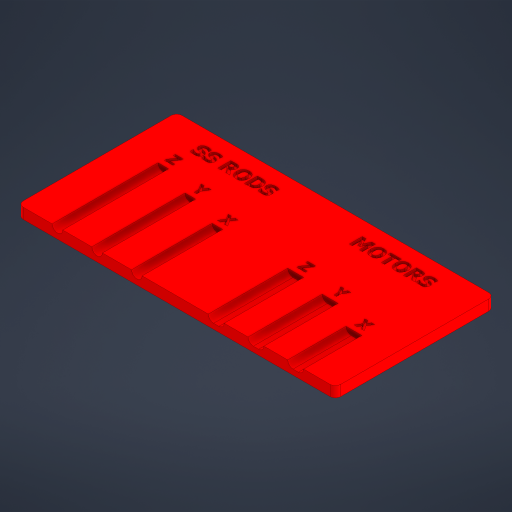
# Autodesk Inventor part: Rod_Motor_Lengths
Saved by Autodesk Inventor 2023.4 (Build 274418000, 418)
## iProperties
Created: 2024-09-24
Part Number: Rod_Motor_Lengths
Material: Generic
Document SubType Name: Modeling
Designer: xSibe
Density: 1 g/cm^3
Appearance: Plastic Red
Author: xSibe
Autodesk Inventor part; units mm, degrees
ref_plane "YZ Plane" through (0, 0, 0) normal (1, 0, 0) x (0, 1, 0)
ref_plane "XZ Plane" through (0, 0, 0) normal (0, 1, 0) x (-1, 0, 0)
ref_plane "XY Plane" through (0, 0, 0) normal (0, 0, 1) x (1, 0, 0)
sketch "Sketch1" plane through (0, 0, 0) normal (0, 1, 0) x (-1, 0, 0)
  line L0 (75, 37.5) -> (-75, 37.5)
  line L1 (-75, 37.5) -> (-75, -37.5)
  line L2 (-75, -37.5) -> (75, -37.5)
  line L3 (75, -37.5) -> (75, 37.5)
  line L4 (75, 37.5) -> (-75, -37.5) construction
  line L5 (-75, 37.5) -> (75, -37.5) construction
  line L6 (0, 37.5) -> (0, -37.5)
  line L7 (0, 37.5) -> (75, 37.5)
  line L8 (0, 37.5) -> (37.5, 37.5)
  line L9 (37.5, 37.5) -> (75, 37.5)
  line L10 (56.25, 37.5) -> (56.25, -12.5)
  line L11 (37.5, 37.5) -> (37.5, -6.5)
  line L12 (18.75, 37.5) -> (18.75, -0.5)
  line L13 (-18.75, 37.5) -> (-18.75, 0)
  line L14 (-37.5, 37.5) -> (-37.5, 2.5)
  line L15 (-56.25, 37.5) -> (-56.25, 10)
  line L16 (58.75, -12.5) -> (53.75, -12.5)
  line L17 (53.75, -12.5) -> (53.75, 37.5)
  line L18 (53.75, 37.5) -> (58.75, 37.5)
  line L19 (58.75, 37.5) -> (58.75, -12.5)
  line L20 (58.75, -12.5) -> (53.75, 37.5) construction
  line L21 (53.75, -12.5) -> (58.75, 37.5) construction
  line L22 (40, -6.5) -> (35, -6.5)
  line L23 (35, -6.5) -> (35, 37.5)
  line L24 (35, 37.5) -> (40, 37.5)
  line L25 (40, 37.5) -> (40, -6.5)
  line L26 (40, -6.5) -> (35, 37.5) construction
  line L27 (35, -6.5) -> (40, 37.5) construction
  line L28 (21.25, -0.5) -> (16.25, -0.5)
  line L29 (16.25, -0.5) -> (16.25, 37.5)
  line L30 (16.25, 37.5) -> (21.25, 37.5)
  line L31 (21.25, 37.5) -> (21.25, -0.5)
  line L32 (21.25, -0.5) -> (16.25, 37.5) construction
  line L33 (16.25, -0.5) -> (21.25, 37.5) construction
  line L34 (0, 37.5) -> (-75, 37.5)
  line L35 (-37.5, 37.5) -> (-75, 37.5)
  line L36 (-37.5, 37.5) -> (0, 37.5)
  line L37 (-15, 0) -> (-22.5, 0)
  line L38 (-22.5, 0) -> (-22.5, 37.5)
  line L39 (-22.5, 37.5) -> (-15, 37.5)
  line L40 (-15, 37.5) -> (-15, 0)
  line L41 (-15, 0) -> (-22.5, 37.5) construction
  line L42 (-22.5, 0) -> (-15, 37.5) construction
  line L43 (-33.75, 2.5) -> (-41.25, 2.5)
  line L44 (-41.25, 2.5) -> (-41.25, 37.5)
  line L45 (-41.25, 37.5) -> (-33.75, 37.5)
  line L46 (-33.75, 37.5) -> (-33.75, 2.5)
  line L47 (-33.75, 2.5) -> (-41.25, 37.5) construction
  line L48 (-41.25, 2.5) -> (-33.75, 37.5) construction
  line L49 (-52.5, 10) -> (-60, 10)
  line L50 (-60, 10) -> (-60, 37.5)
  line L51 (-60, 37.5) -> (-52.5, 37.5)
  line L52 (-52.5, 37.5) -> (-52.5, 10)
  line L53 (-52.5, 10) -> (-60, 37.5) construction
  line L54 (-60, 10) -> (-52.5, 37.5) construction
  point P0 (0, 0)
  point P1 (56.25, 12.5)
  point P2 (37.5, 15.5)
  point P3 (18.75, 18.5)
  point P4 (-18.75, 18.75)
  point P5 (-37.5, 20)
  point P6 (-56.25, 23.75)
  dimension "d0" = 150
  dimension "d1" = 75
  dimension "d2" = 50
  dimension "d3" = 44
  dimension "d4" = 38
  dimension "d5" = 37.5
  dimension "d6" = 35
  dimension "d7" = 27.5
  dimension "d8" = 5
  dimension "d9" = 5
  dimension "d10" = 5
  dimension "d11" = 7.5
  dimension "d12" = 7.5
  dimension "d13" = 7.5
  constraints: 110 end point, 28 midpoint, 14 parallel, 12 perpendicular, 7 horizontal, 6 point on line, 4 vertical, 3 collinear
  measures "d0" distance of L2.end L1.end
  measures "d1" distance of L1.end L0.end
  measures "d2" distance of L10.start L10.end
  measures "d3" distance of L8.end L11.end
  measures "d4" distance of L12.start L12.end
  measures "d5" distance of L13.start L13.end
  measures "d6" distance of L14.start L14.end
  measures "d7" distance of L15.start L15.end
  measures "d8" distance of L17.end L18.end
  measures "d9" distance of L23.end L24.end
  measures "d10" distance of L29.end L30.end
  measures "d11" distance of L38.end L39.end
  measures "d12" distance of L44.end L45.end
  measures "d13" distance of L50.end L51.end
extrude "Extrusion1" add sketch "Sketch1" along normal blind 5 contours L3 L2 L6 L0 L29 L28 L31 L23 L22 L25 L17 L16 L19 | L2 L1 L0 L50 L49 L52 L44 L43 L46 L38 L37 L40 L6
extrude "Extrusion2" add sketch "Sketch1" along normal blind 2.5
sketch "Sketch2" plane through (0, 5, 0) normal (0, 1, 0) x (1, 0, 0)
  line L0 (-75, -37.5) -> (-58.75, -37.5) projected
  line L1 (-58.75, -37.5) -> (-58.75, 12.5) projected
  line L2 (-58.75, 12.5) -> (-53.75, 12.5) projected
  line L3 (-53.75, 12.5) -> (-53.75, -37.5) projected
  line L4 (-53.75, -37.5) -> (-40, -37.5) projected
  line L5 (-40, -37.5) -> (-40, 6.5) projected
  line L6 (-40, 6.5) -> (-35, 6.5) projected
  line L7 (-35, 6.5) -> (-35, -37.5) projected
  line L8 (-35, -37.5) -> (-21.25, -37.5) projected
  line L9 (-21.25, -37.5) -> (-21.25, 0.5) projected
  line L10 (-21.25, 0.5) -> (-16.25, 0.5) projected
  line L11 (-16.25, 0.5) -> (-16.25, -37.5) projected
  line L12 (-16.25, -37.5) -> (15, -37.5) projected
  line L13 (15, -37.5) -> (15, 0) projected
  line L14 (15, 0) -> (22.5, 0) projected
  line L15 (22.5, 0) -> (22.5, -37.5) projected
  line L16 (22.5, -37.5) -> (33.75, -37.5) projected
  line L17 (33.75, -37.5) -> (33.75, -2.5) projected
  line L18 (33.75, -2.5) -> (41.25, -2.5) projected
  line L19 (41.25, -2.5) -> (41.25, -37.5) projected
  line L20 (41.25, -37.5) -> (52.5, -37.5) projected
  line L21 (52.5, -37.5) -> (52.5, -10) projected
  line L22 (52.5, -10) -> (60, -10) projected
  line L23 (60, -10) -> (60, -37.5) projected
  line L24 (60, -37.5) -> (75, -37.5) projected
  line L25 (75, -37.5) -> (75, 37.5) projected
  line L26 (75, 37.5) -> (-75, 37.5) projected
  line L27 (-75, 37.5) -> (-75, -37.5) projected
  line L28 (-75, 37.5) -> (0, 37.5)
  line L29 (0, 37.5) -> (0, 0)
  line L30 (0, 0) -> (-75, 0)
  line L31 (-75, 0) -> (-75, 37.5)
  line L32 (0, 37.5) -> (75, 37.5)
  line L33 (75, 37.5) -> (75, 0)
  line L34 (75, 0) -> (0, 0)
  line L35 (0, 0) -> (0, 37.5)
  line L36 (-37.5, 37.5) -> (-37.5, 27.5)
  line L37 (-62.5, 22.5) -> (-12.5, 22.5)
  line L38 (-12.5, 22.5) -> (-12.5, 32.5)
  line L39 (-12.5, 32.5) -> (-62.5, 32.5)
  line L40 (-62.5, 32.5) -> (-62.5, 22.5)
  line L41 (-62.5, 22.5) -> (-12.5, 32.5) construction
  line L42 (-12.5, 22.5) -> (-62.5, 32.5) construction
  line L43 (37.5, 37.5) -> (37.5, 27.5)
  line L44 (12.5, 22.5) -> (62.5, 22.5)
  line L45 (62.5, 22.5) -> (62.5, 32.5)
  line L46 (62.5, 32.5) -> (12.5, 32.5)
  line L47 (12.5, 32.5) -> (12.5, 22.5)
  line L48 (12.5, 22.5) -> (62.5, 32.5) construction
  line L49 (62.5, 22.5) -> (12.5, 32.5) construction
  line L50 (-62.5, 32.5) -> (-12.5, 32.5) construction
  line L51 (-12.5, 32.5) -> (-12.5, 22.5) construction
  line L52 (-12.5, 22.5) -> (-62.5, 22.5) construction
  line L53 (-62.5, 22.5) -> (-62.5, 32.5) construction
  line L54 (12.5, 32.5) -> (62.5, 32.5) construction
  line L55 (62.5, 32.5) -> (62.5, 22.5) construction
  line L56 (62.5, 22.5) -> (12.5, 22.5) construction
  line L57 (12.5, 22.5) -> (12.5, 32.5) construction
  line L58 (-58.75, 20) -> (-53.75, 20) construction
  line L59 (-53.75, 20) -> (-53.75, 12.5) construction
  line L60 (-53.75, 12.5) -> (-58.75, 12.5) construction
  line L61 (-58.75, 12.5) -> (-58.75, 20) construction
  line L62 (-40, 14) -> (-35, 14) construction
  line L63 (-35, 14) -> (-35, 6.5) construction
  line L64 (-35, 6.5) -> (-40, 6.5) construction
  line L65 (-40, 6.5) -> (-40, 14) construction
  line L66 (-21.25, 8) -> (-16.25, 8) construction
  line L67 (-16.25, 8) -> (-16.25, 0.5) construction
  line L68 (-16.25, 0.5) -> (-21.25, 0.5) construction
  line L69 (-21.25, 0.5) -> (-21.25, 8) construction
  line L70 (15, 7.5) -> (22.5, 7.5) construction
  line L71 (22.5, 7.5) -> (22.5, 0) construction
  line L72 (22.5, 0) -> (15, 0) construction
  line L73 (15, 0) -> (15, 7.5) construction
  line L74 (33.75, 5) -> (41.25, 5) construction
  line L75 (41.25, 5) -> (41.25, -2.5) construction
  line L76 (41.25, -2.5) -> (33.75, -2.5) construction
  line L77 (33.75, -2.5) -> (33.75, 5) construction
  line L78 (52.5, -2.5) -> (60, -2.5) construction
  line L79 (60, -2.5) -> (60, -10) construction
  line L80 (60, -10) -> (52.5, -10) construction
  line L81 (52.5, -10) -> (52.5, -2.5) construction
  spline S0 degree 2 poles (-53.6348, 24.3412) (-54.3368, 24.3412) (-55.3947, 24.6131) (-55.8494, 24.8109) knots 0 0 0 1 2 2 2
  line L82 (-55.8494, 24.8109) -> (-55.8494, 26.2642)
  line L83 (-55.8494, 26.2642) -> (-55.711, 26.2642)
  spline S1 degree 2 poles (-55.711, 26.2642) (-55.2513, 25.8737) (-54.1489, 25.4535) (-53.6299, 25.4535) knots 0 0 0 1 2 2 2
  spline S2 degree 2 poles (-53.6299, 25.4535) (-53.4964, 25.4535) (-53.0664, 25.5128) (-52.9378, 25.5721) knots 0 0 0 1 2 2 2
  spline S3 degree 2 poles (-52.9378, 25.5721) (-52.7797, 25.6413) (-52.5572, 25.8934) (-52.5572, 26.0961) knots 0 0 0 1 2 2 2
  spline S4 degree 2 poles (-52.5572, 26.0961) (-52.5572, 26.3284) (-52.9181, 26.6152) (-53.1652, 26.6794) knots 0 0 0 1 2 2 2
  spline S5 degree 2 poles (-53.1652, 26.6794) (-53.4767, 26.7635) (-54.1835, 26.9068) (-54.495, 27.0156) knots 0 0 0 1 2 2 2
  spline S6 degree 2 poles (-54.495, 27.0156) (-55.2019, 27.2627) (-55.8148, 28.108) (-55.8148, 28.7408) knots 0 0 0 1 2 2 2
  spline S7 degree 2 poles (-55.8148, 28.7408) (-55.8148, 29.5959) (-54.3665, 30.6588) (-53.2789, 30.6588) knots 0 0 0 1 2 2 2
  spline S8 degree 2 poles (-53.2789, 30.6588) (-52.7352, 30.6588) (-51.6575, 30.4363) (-51.2324, 30.2485) knots 0 0 0 1 2 2 2
  line L84 (-51.2324, 30.2485) -> (-51.2324, 28.8545)
  line L85 (-51.2324, 28.8545) -> (-51.3659, 28.8545)
  spline S9 degree 2 poles (-51.3659, 28.8545) (-51.707, 29.1461) (-52.6857, 29.5465) (-53.1998, 29.5465) knots 0 0 0 1 2 2 2
  spline S10 degree 2 poles (-53.1998, 29.5465) (-53.4025, 29.5465) (-53.7189, 29.4872) (-53.8968, 29.4081) knots 0 0 0 1 2 2 2
  spline S11 degree 2 poles (-53.8968, 29.4081) (-54.0402, 29.3438) (-54.2478, 29.0868) (-54.2478, 28.9286) knots 0 0 0 1 2 2 2
  spline S12 degree 2 poles (-54.2478, 28.9286) (-54.2478, 28.6913) (-53.9166, 28.4194) (-53.4421, 28.3107) knots 0 0 0 1 2 2 2
  spline S13 degree 2 poles (-53.4421, 28.3107) (-53.1356, 28.2415) (-52.5671, 28.108) (-52.2408, 27.9943) knots 0 0 0 1 2 2 2
  spline S14 degree 2 poles (-52.2408, 27.9943) (-51.6081, 27.762) (-50.9902, 26.9908) (-50.9902, 26.3581) knots 0 0 0 1 2 2 2
  spline S15 degree 2 poles (-50.9902, 26.3581) (-50.9902, 25.4485) (-52.4188, 24.3412) (-53.6348, 24.3412) knots 0 0 0 1 2 2 2
  spline S16 degree 2 poles (-48.3208, 24.3412) (-49.0228, 24.3412) (-50.0806, 24.6131) (-50.5354, 24.8109) knots 0 0 0 1 2 2 2
  line L86 (-50.5354, 24.8109) -> (-50.5354, 26.2642)
  line L87 (-50.5354, 26.2642) -> (-50.397, 26.2642)
  spline S17 degree 2 poles (-50.397, 26.2642) (-49.9373, 25.8737) (-48.8349, 25.4535) (-48.3159, 25.4535) knots 0 0 0 1 2 2 2
  spline S18 degree 2 poles (-48.3159, 25.4535) (-48.1824, 25.4535) (-47.7524, 25.5128) (-47.6238, 25.5721) knots 0 0 0 1 2 2 2
  spline S19 degree 2 poles (-47.6238, 25.5721) (-47.4656, 25.6413) (-47.2432, 25.8934) (-47.2432, 26.0961) knots 0 0 0 1 2 2 2
  spline S20 degree 2 poles (-47.2432, 26.0961) (-47.2432, 26.3284) (-47.6041, 26.6152) (-47.8512, 26.6794) knots 0 0 0 1 2 2 2
  spline S21 degree 2 poles (-47.8512, 26.6794) (-48.1626, 26.7635) (-48.8695, 26.9068) (-49.181, 27.0156) knots 0 0 0 1 2 2 2
  spline S22 degree 2 poles (-49.181, 27.0156) (-49.8878, 27.2627) (-50.5008, 28.108) (-50.5008, 28.7408) knots 0 0 0 1 2 2 2
  spline S23 degree 2 poles (-50.5008, 28.7408) (-50.5008, 29.5959) (-49.0524, 30.6588) (-47.9649, 30.6588) knots 0 0 0 1 2 2 2
  spline S24 degree 2 poles (-47.9649, 30.6588) (-47.4212, 30.6588) (-46.3435, 30.4363) (-45.9184, 30.2485) knots 0 0 0 1 2 2 2
  line L88 (-45.9184, 30.2485) -> (-45.9184, 28.8545)
  line L89 (-45.9184, 28.8545) -> (-46.0519, 28.8545)
  spline S25 degree 2 poles (-46.0519, 28.8545) (-46.3929, 29.1461) (-47.3717, 29.5465) (-47.8858, 29.5465) knots 0 0 0 1 2 2 2
  spline S26 degree 2 poles (-47.8858, 29.5465) (-48.0885, 29.5465) (-48.4049, 29.4872) (-48.5828, 29.4081) knots 0 0 0 1 2 2 2
  spline S27 degree 2 poles (-48.5828, 29.4081) (-48.7262, 29.3438) (-48.9338, 29.0868) (-48.9338, 28.9286) knots 0 0 0 1 2 2 2
  spline S28 degree 2 poles (-48.9338, 28.9286) (-48.9338, 28.6913) (-48.6026, 28.4194) (-48.128, 28.3107) knots 0 0 0 1 2 2 2
  spline S29 degree 2 poles (-48.128, 28.3107) (-47.8216, 28.2415) (-47.2531, 28.108) (-46.9268, 27.9943) knots 0 0 0 1 2 2 2
  spline S30 degree 2 poles (-46.9268, 27.9943) (-46.2941, 27.762) (-45.6762, 26.9908) (-45.6762, 26.3581) knots 0 0 0 1 2 2 2
  spline S31 degree 2 poles (-45.6762, 26.3581) (-45.6762, 25.4485) (-47.1048, 24.3412) (-48.3208, 24.3412) knots 0 0 0 1 2 2 2
  line L90 (-36.7981, 24.45) -> (-38.6617, 24.45)
  line L91 (-38.6617, 24.45) -> (-40.3572, 26.6893)
  line L92 (-40.3572, 26.6893) -> (-40.9109, 26.6893)
  line L93 (-40.9109, 26.6893) -> (-40.9109, 24.45)
  line L94 (-40.9109, 24.45) -> (-42.4334, 24.45)
  line L95 (-42.4334, 24.45) -> (-42.4334, 30.55)
  line L96 (-42.4334, 30.55) -> (-39.9815, 30.55)
  spline S32 degree 2 poles (-39.9815, 30.55) (-39.4724, 30.55) (-38.721, 30.4215) (-38.3997, 30.2237) knots 0 0 0 1 2 2 2
  spline S33 degree 2 poles (-38.3997, 30.2237) (-38.0734, 30.0161) (-37.6878, 29.3686) (-37.6878, 28.8742) knots 0 0 0 1 2 2 2
  spline S34 degree 2 poles (-37.6878, 28.8742) (-37.6878, 28.1772) (-38.3206, 27.3023) (-38.8495, 27.0452) knots 0 0 0 1 2 2 2
  line L97 (-38.8495, 27.0452) -> (-36.7981, 24.45)
  spline S35 degree 2 poles (-39.2598, 28.6814) (-39.2598, 28.9138) (-39.4378, 29.245) (-39.6404, 29.334) knots 0 0 0 1 2 2 2
  spline S36 degree 2 poles (-39.6404, 29.334) (-39.7838, 29.3933) (-40.1348, 29.4279) (-40.3968, 29.4279) knots 0 0 0 1 2 2 2
  line L98 (-40.3968, 29.4279) -> (-40.9109, 29.4279)
  line L99 (-40.9109, 29.4279) -> (-40.9109, 27.7867)
  line L100 (-40.9109, 27.7867) -> (-40.4709, 27.7867)
  spline S37 degree 2 poles (-40.4709, 27.7867) (-40.1545, 27.7867) (-39.7047, 27.8658) (-39.5515, 27.9894) knots 0 0 0 1 2 2 2
  spline S38 degree 2 poles (-39.5515, 27.9894) (-39.4032, 28.108) (-39.2598, 28.4244) (-39.2598, 28.6814) knots 0 0 0 1 2 2 2
  spline S39 degree 2 poles (-30.792, 27.5) (-30.792, 26.017) (-32.3738, 24.3215) (-33.7481, 24.3215) knots 0 0 0 1 2 2 2
  spline S40 degree 2 poles (-33.7481, 24.3215) (-35.1272, 24.3215) (-36.6992, 26.0368) (-36.6992, 27.5) knots 0 0 0 1 2 2 2
  spline S41 degree 2 poles (-36.6992, 27.5) (-36.6992, 28.9682) (-35.1272, 30.6785) (-33.7481, 30.6785) knots 0 0 0 1 2 2 2
  spline S42 degree 2 poles (-33.7481, 30.6785) (-32.3738, 30.6785) (-30.792, 28.978) (-30.792, 27.5) knots 0 0 0 1 2 2 2
  spline S43 degree 2 poles (-32.3738, 27.5) (-32.3738, 28.0487) (-32.5963, 28.8149) (-32.7891, 29.0571) knots 0 0 0 1 2 2 2
  spline S44 degree 2 poles (-32.7891, 29.0571) (-32.9818, 29.3092) (-33.4762, 29.5267) (-33.7431, 29.5267) knots 0 0 0 1 2 2 2
  spline S45 degree 2 poles (-33.7431, 29.5267) (-34.0249, 29.5267) (-34.4846, 29.3241) (-34.6972, 29.067) knots 0 0 0 1 2 2 2
  spline S46 degree 2 poles (-34.6972, 29.067) (-34.885, 28.8297) (-35.1173, 28.0438) (-35.1173, 27.5) knots 0 0 0 1 2 2 2
  spline S47 degree 2 poles (-35.1173, 27.5) (-35.1173, 26.9365) (-34.8949, 26.195) (-34.7021, 25.9429) knots 0 0 0 1 2 2 2
  spline S48 degree 2 poles (-34.7021, 25.9429) (-34.5093, 25.6908) (-34.01, 25.4733) (-33.7431, 25.4733) knots 0 0 0 1 2 2 2
  spline S49 degree 2 poles (-33.7431, 25.4733) (-33.4712, 25.4733) (-32.967, 25.7056) (-32.7841, 25.9528) knots 0 0 0 1 2 2 2
  spline S50 degree 2 poles (-32.7841, 25.9528) (-32.5864, 26.2197) (-32.3738, 26.9266) (-32.3738, 27.5) knots 0 0 0 1 2 2 2
  spline S51 degree 2 poles (-24.4399, 27.4951) (-24.4399, 26.6399) (-25.1863, 25.2953) (-25.7548, 24.9344) knots 0 0 0 1 2 2 2
  spline S52 degree 2 poles (-25.7548, 24.9344) (-26.2293, 24.628) (-27.3465, 24.45) (-27.9743, 24.45) knots 0 0 0 1 2 2 2
  line L101 (-27.9743, 24.45) -> (-29.8824, 24.45)
  line L102 (-29.8824, 24.45) -> (-29.8824, 30.55)
  line L103 (-29.8824, 30.55) -> (-27.9941, 30.55)
  spline S53 degree 2 poles (-27.9941, 30.55) (-27.3515, 30.55) (-26.2293, 30.3869) (-25.735, 30.0705) knots 0 0 0 1 2 2 2
  spline S54 degree 2 poles (-25.735, 30.0705) (-25.1369, 29.6849) (-24.4399, 28.3799) (-24.4399, 27.4951) knots 0 0 0 1 2 2 2
  spline S55 degree 2 poles (-26.0118, 27.5049) (-26.0118, 28.108) (-26.4271, 28.9682) (-26.8522, 29.2104) knots 0 0 0 1 2 2 2
  spline S56 degree 2 poles (-26.8522, 29.2104) (-27.1636, 29.3784) (-27.8458, 29.413) (-28.3203, 29.413) knots 0 0 0 1 2 2 2
  line L104 (-28.3203, 29.413) -> (-28.35, 29.413)
  line L105 (-28.35, 29.413) -> (-28.35, 25.5919)
  line L106 (-28.35, 25.5919) -> (-28.3203, 25.5919)
  spline S57 degree 2 poles (-28.3203, 25.5919) (-27.8062, 25.5919) (-27.0994, 25.6265) (-26.778, 25.8292) knots 0 0 0 1 2 2 2
  spline S58 degree 2 poles (-26.778, 25.8292) (-26.4023, 26.0665) (-26.0118, 26.9019) (-26.0118, 27.5049) knots 0 0 0 1 2 2 2
  spline S59 degree 2 poles (-21.6469, 24.3412) (-22.3489, 24.3412) (-23.4067, 24.6131) (-23.8615, 24.8109) knots 0 0 0 1 2 2 2
  line L107 (-23.8615, 24.8109) -> (-23.8615, 26.2642)
  line L108 (-23.8615, 26.2642) -> (-23.7231, 26.2642)
  spline S60 degree 2 poles (-23.7231, 26.2642) (-23.2634, 25.8737) (-22.161, 25.4535) (-21.642, 25.4535) knots 0 0 0 1 2 2 2
  spline S61 degree 2 poles (-21.642, 25.4535) (-21.5085, 25.4535) (-21.0784, 25.5128) (-20.9499, 25.5721) knots 0 0 0 1 2 2 2
  spline S62 degree 2 poles (-20.9499, 25.5721) (-20.7917, 25.6413) (-20.5693, 25.8934) (-20.5693, 26.0961) knots 0 0 0 1 2 2 2
  spline S63 degree 2 poles (-20.5693, 26.0961) (-20.5693, 26.3284) (-20.9301, 26.6152) (-21.1773, 26.6794) knots 0 0 0 1 2 2 2
  spline S64 degree 2 poles (-21.1773, 26.6794) (-21.4887, 26.7635) (-22.1956, 26.9068) (-22.507, 27.0156) knots 0 0 0 1 2 2 2
  spline S65 degree 2 poles (-22.507, 27.0156) (-23.2139, 27.2627) (-23.8269, 28.108) (-23.8269, 28.7408) knots 0 0 0 1 2 2 2
  spline S66 degree 2 poles (-23.8269, 28.7408) (-23.8269, 29.5959) (-22.3785, 30.6588) (-21.291, 30.6588) knots 0 0 0 1 2 2 2
  spline S67 degree 2 poles (-21.291, 30.6588) (-20.7472, 30.6588) (-19.6696, 30.4363) (-19.2445, 30.2485) knots 0 0 0 1 2 2 2
  line L109 (-19.2445, 30.2485) -> (-19.2445, 28.8545)
  line L110 (-19.2445, 28.8545) -> (-19.378, 28.8545)
  spline S68 degree 2 poles (-19.378, 28.8545) (-19.719, 29.1461) (-20.6978, 29.5465) (-21.2119, 29.5465) knots 0 0 0 1 2 2 2
  spline S69 degree 2 poles (-21.2119, 29.5465) (-21.4146, 29.5465) (-21.731, 29.4872) (-21.9089, 29.4081) knots 0 0 0 1 2 2 2
  spline S70 degree 2 poles (-21.9089, 29.4081) (-22.0523, 29.3438) (-22.2599, 29.0868) (-22.2599, 28.9286) knots 0 0 0 1 2 2 2
  spline S71 degree 2 poles (-22.2599, 28.9286) (-22.2599, 28.6913) (-21.9287, 28.4194) (-21.4541, 28.3107) knots 0 0 0 1 2 2 2
  spline S72 degree 2 poles (-21.4541, 28.3107) (-21.1476, 28.2415) (-20.5792, 28.108) (-20.2529, 27.9943) knots 0 0 0 1 2 2 2
  spline S73 degree 2 poles (-20.2529, 27.9943) (-19.6202, 27.762) (-19.0023, 26.9908) (-19.0023, 26.3581) knots 0 0 0 1 2 2 2
  spline S74 degree 2 poles (-19.0023, 26.3581) (-19.0023, 25.4485) (-20.4309, 24.3412) (-21.6469, 24.3412) knots 0 0 0 1 2 2 2
  line L111 (-54.2443, 15) -> (-58.2071, 15)
  line L112 (-58.2071, 15) -> (-58.2071, 15.936)
  line L113 (-58.2071, 15.936) -> (-55.9015, 19.0478)
  line L114 (-55.9015, 19.0478) -> (-58.0855, 19.0478)
  line L115 (-58.0855, 19.0478) -> (-58.0855, 20)
  line L116 (-58.0855, 20) -> (-54.378, 20)
  line L117 (-54.378, 20) -> (-54.378, 19.0478)
  line L118 (-54.378, 19.0478) -> (-56.6754, 15.9522)
  line L119 (-56.6754, 15.9522) -> (-54.2443, 15.9522)
  line L120 (-54.2443, 15.9522) -> (-54.2443, 15)
  line L121 (-35.1925, 14) -> (-36.9186, 11.0867)
  line L122 (-36.9186, 11.0867) -> (-36.9186, 9)
  line L123 (-36.9186, 9) -> (-38.1746, 9)
  line L124 (-38.1746, 9) -> (-38.1746, 11.0259)
  line L125 (-38.1746, 11.0259) -> (-39.9291, 14)
  line L126 (-39.9291, 14) -> (-38.4988, 14)
  line L127 (-38.4988, 14) -> (-37.5223, 12.2172)
  line L128 (-37.5223, 12.2172) -> (-36.5782, 14)
  line L129 (-36.5782, 14) -> (-35.1925, 14)
  line L130 (-16.3959, 3) -> (-17.8464, 3)
  line L131 (-17.8464, 3) -> (-18.8108, 4.5924)
  line L132 (-18.8108, 4.5924) -> (-19.7954, 3)
  line L133 (-19.7954, 3) -> (-21.1852, 3)
  line L134 (-21.1852, 3) -> (-19.5604, 5.5162)
  line L135 (-19.5604, 5.5162) -> (-21.1203, 8)
  line L136 (-21.1203, 8) -> (-19.6698, 8)
  line L137 (-19.6698, 8) -> (-18.7662, 6.4887)
  line L138 (-18.7662, 6.4887) -> (-17.8383, 8)
  line L139 (-17.8383, 8) -> (-16.4485, 8)
  line L140 (-16.4485, 8) -> (-18.0166, 5.5689)
  line L141 (-18.0166, 5.5689) -> (-16.3959, 3)
  line L142 (20.7557, 2.5) -> (16.7929, 2.5)
  line L143 (16.7929, 2.5) -> (16.7929, 3.436)
  line L144 (16.7929, 3.436) -> (19.0985, 6.5478)
  line L145 (19.0985, 6.5478) -> (16.9145, 6.5478)
  line L146 (16.9145, 6.5478) -> (16.9145, 7.5)
  line L147 (16.9145, 7.5) -> (20.622, 7.5)
  line L148 (20.622, 7.5) -> (20.622, 6.5478)
  line L149 (20.622, 6.5478) -> (18.3246, 3.4522)
  line L150 (18.3246, 3.4522) -> (20.7557, 3.4522)
  line L151 (20.7557, 3.4522) -> (20.7557, 2.5)
  line L152 (25.8833, 24.45) -> (24.3608, 24.45)
  line L153 (24.3608, 24.45) -> (24.3608, 28.4936)
  line L154 (24.3608, 28.4936) -> (23.2535, 25.8835)
  line L155 (23.2535, 25.8835) -> (22.2055, 25.8835)
  line L156 (22.2055, 25.8835) -> (21.0982, 28.4936)
  line L157 (21.0982, 28.4936) -> (21.0982, 24.45)
  line L158 (21.0982, 24.45) -> (19.6548, 24.45)
  line L159 (19.6548, 24.45) -> (19.6548, 30.55)
  line L160 (19.6548, 30.55) -> (21.4195, 30.55)
  line L161 (21.4195, 30.55) -> (22.774, 27.5395)
  line L162 (22.774, 27.5395) -> (24.1186, 30.55)
  line L163 (24.1186, 30.55) -> (25.8833, 30.55)
  line L164 (25.8833, 30.55) -> (25.8833, 24.45)
  spline S75 degree 2 poles (32.7001, 27.5) (32.7001, 26.017) (31.1182, 24.3215) (29.744, 24.3215) knots 0 0 0 1 2 2 2
  spline S76 degree 2 poles (29.744, 24.3215) (28.3648, 24.3215) (26.7929, 26.0368) (26.7929, 27.5) knots 0 0 0 1 2 2 2
  spline S77 degree 2 poles (26.7929, 27.5) (26.7929, 28.9682) (28.3648, 30.6785) (29.744, 30.6785) knots 0 0 0 1 2 2 2
  spline S78 degree 2 poles (29.744, 30.6785) (31.1182, 30.6785) (32.7001, 28.978) (32.7001, 27.5) knots 0 0 0 1 2 2 2
  spline S79 degree 2 poles (31.1182, 27.5) (31.1182, 28.0487) (30.8958, 28.8149) (30.703, 29.0571) knots 0 0 0 1 2 2 2
  spline S80 degree 2 poles (30.703, 29.0571) (30.5102, 29.3092) (30.0159, 29.5267) (29.7489, 29.5267) knots 0 0 0 1 2 2 2
  spline S81 degree 2 poles (29.7489, 29.5267) (29.4672, 29.5267) (29.0075, 29.3241) (28.7949, 29.067) knots 0 0 0 1 2 2 2
  spline S82 degree 2 poles (28.7949, 29.067) (28.607, 28.8297) (28.3747, 28.0438) (28.3747, 27.5) knots 0 0 0 1 2 2 2
  spline S83 degree 2 poles (28.3747, 27.5) (28.3747, 26.9365) (28.5972, 26.195) (28.79, 25.9429) knots 0 0 0 1 2 2 2
  spline S84 degree 2 poles (28.79, 25.9429) (28.9827, 25.6908) (29.482, 25.4733) (29.7489, 25.4733) knots 0 0 0 1 2 2 2
  spline S85 degree 2 poles (29.7489, 25.4733) (30.0208, 25.4733) (30.525, 25.7056) (30.7079, 25.9528) knots 0 0 0 1 2 2 2
  spline S86 degree 2 poles (30.7079, 25.9528) (30.9057, 26.2197) (31.1182, 26.9266) (31.1182, 27.5) knots 0 0 0 1 2 2 2
  line L165 (34.7812, 24.45) -> (34.7812, 29.3883)
  line L166 (34.7812, 29.3883) -> (32.9769, 29.3883)
  line L167 (32.9769, 29.3883) -> (32.9769, 30.55)
  line L168 (32.9769, 30.55) -> (38.1179, 30.55)
  line L169 (38.1179, 30.55) -> (38.1179, 29.3883)
  line L170 (38.1179, 29.3883) -> (36.3136, 29.3883)
  line L171 (36.3136, 29.3883) -> (36.3136, 24.45)
  line L172 (36.3136, 24.45) -> (34.7812, 24.45)
  spline S87 degree 2 poles (44.297, 27.5) (44.297, 26.017) (42.7152, 24.3215) (41.3409, 24.3215) knots 0 0 0 1 2 2 2
  spline S88 degree 2 poles (41.3409, 24.3215) (39.9618, 24.3215) (38.3898, 26.0368) (38.3898, 27.5) knots 0 0 0 1 2 2 2
  spline S89 degree 2 poles (38.3898, 27.5) (38.3898, 28.9682) (39.9618, 30.6785) (41.3409, 30.6785) knots 0 0 0 1 2 2 2
  spline S90 degree 2 poles (41.3409, 30.6785) (42.7152, 30.6785) (44.297, 28.978) (44.297, 27.5) knots 0 0 0 1 2 2 2
  spline S91 degree 2 poles (42.7152, 27.5) (42.7152, 28.0487) (42.4927, 28.8149) (42.2999, 29.0571) knots 0 0 0 1 2 2 2
  spline S92 degree 2 poles (42.2999, 29.0571) (42.1071, 29.3092) (41.6128, 29.5267) (41.3459, 29.5267) knots 0 0 0 1 2 2 2
  spline S93 degree 2 poles (41.3459, 29.5267) (41.0641, 29.5267) (40.6044, 29.3241) (40.3918, 29.067) knots 0 0 0 1 2 2 2
  spline S94 degree 2 poles (40.3918, 29.067) (40.204, 28.8297) (39.9716, 28.0438) (39.9716, 27.5) knots 0 0 0 1 2 2 2
  spline S95 degree 2 poles (39.9716, 27.5) (39.9716, 26.9365) (40.1941, 26.195) (40.3869, 25.9429) knots 0 0 0 1 2 2 2
  spline S96 degree 2 poles (40.3869, 25.9429) (40.5797, 25.6908) (41.0789, 25.4733) (41.3459, 25.4733) knots 0 0 0 1 2 2 2
  spline S97 degree 2 poles (41.3459, 25.4733) (41.6177, 25.4733) (42.122, 25.7056) (42.3049, 25.9528) knots 0 0 0 1 2 2 2
  spline S98 degree 2 poles (42.3049, 25.9528) (42.5026, 26.2197) (42.7152, 26.9266) (42.7152, 27.5) knots 0 0 0 1 2 2 2
  line L173 (50.8419, 24.45) -> (48.9783, 24.45)
  line L174 (48.9783, 24.45) -> (47.2827, 26.6893)
  line L175 (47.2827, 26.6893) -> (46.7291, 26.6893)
  line L176 (46.7291, 26.6893) -> (46.7291, 24.45)
  line L177 (46.7291, 24.45) -> (45.2066, 24.45)
  line L178 (45.2066, 24.45) -> (45.2066, 30.55)
  line L179 (45.2066, 30.55) -> (47.6584, 30.55)
  spline S99 degree 2 poles (47.6584, 30.55) (48.1676, 30.55) (48.919, 30.4215) (49.2403, 30.2237) knots 0 0 0 1 2 2 2
  spline S100 degree 2 poles (49.2403, 30.2237) (49.5665, 30.0161) (49.9521, 29.3686) (49.9521, 28.8742) knots 0 0 0 1 2 2 2
  spline S101 degree 2 poles (49.9521, 28.8742) (49.9521, 28.1772) (49.3194, 27.3023) (48.7904, 27.0452) knots 0 0 0 1 2 2 2
  line L180 (48.7904, 27.0452) -> (50.8419, 24.45)
  spline S102 degree 2 poles (48.3801, 28.6814) (48.3801, 28.9138) (48.2022, 29.245) (47.9995, 29.334) knots 0 0 0 1 2 2 2
  spline S103 degree 2 poles (47.9995, 29.334) (47.8562, 29.3933) (47.5052, 29.4279) (47.2432, 29.4279) knots 0 0 0 1 2 2 2
  line L181 (47.2432, 29.4279) -> (46.7291, 29.4279)
  line L182 (46.7291, 29.4279) -> (46.7291, 27.7867)
  line L183 (46.7291, 27.7867) -> (47.169, 27.7867)
  spline S104 degree 2 poles (47.169, 27.7867) (47.4854, 27.7867) (47.9353, 27.8658) (48.0885, 27.9894) knots 0 0 0 1 2 2 2
  spline S105 degree 2 poles (48.0885, 27.9894) (48.2368, 28.108) (48.3801, 28.4244) (48.3801, 28.6814) knots 0 0 0 1 2 2 2
  spline S106 degree 2 poles (53.1801, 24.3412) (52.4781, 24.3412) (51.4203, 24.6131) (50.9655, 24.8109) knots 0 0 0 1 2 2 2
  line L184 (50.9655, 24.8109) -> (50.9655, 26.2642)
  line L185 (50.9655, 26.2642) -> (51.1039, 26.2642)
  spline S107 degree 2 poles (51.1039, 26.2642) (51.5636, 25.8737) (52.666, 25.4535) (53.185, 25.4535) knots 0 0 0 1 2 2 2
  spline S108 degree 2 poles (53.185, 25.4535) (53.3185, 25.4535) (53.7485, 25.5128) (53.8771, 25.5721) knots 0 0 0 1 2 2 2
  spline S109 degree 2 poles (53.8771, 25.5721) (54.0353, 25.6413) (54.2577, 25.8934) (54.2577, 26.0961) knots 0 0 0 1 2 2 2
  spline S110 degree 2 poles (54.2577, 26.0961) (54.2577, 26.3284) (53.8968, 26.6152) (53.6497, 26.6794) knots 0 0 0 1 2 2 2
  spline S111 degree 2 poles (53.6497, 26.6794) (53.3382, 26.7635) (52.6314, 26.9068) (52.3199, 27.0156) knots 0 0 0 1 2 2 2
  spline S112 degree 2 poles (52.3199, 27.0156) (51.613, 27.2627) (51.0001, 28.108) (51.0001, 28.7408) knots 0 0 0 1 2 2 2
  spline S113 degree 2 poles (51.0001, 28.7408) (51.0001, 29.5959) (52.4485, 30.6588) (53.536, 30.6588) knots 0 0 0 1 2 2 2
  spline S114 degree 2 poles (53.536, 30.6588) (54.0797, 30.6588) (55.1574, 30.4363) (55.5825, 30.2485) knots 0 0 0 1 2 2 2
  line L186 (55.5825, 30.2485) -> (55.5825, 28.8545)
  line L187 (55.5825, 28.8545) -> (55.449, 28.8545)
  spline S115 degree 2 poles (55.449, 28.8545) (55.1079, 29.1461) (54.1292, 29.5465) (53.6151, 29.5465) knots 0 0 0 1 2 2 2
  spline S116 degree 2 poles (53.6151, 29.5465) (53.4124, 29.5465) (53.096, 29.4872) (52.9181, 29.4081) knots 0 0 0 1 2 2 2
  spline S117 degree 2 poles (52.9181, 29.4081) (52.7747, 29.3438) (52.5671, 29.0868) (52.5671, 28.9286) knots 0 0 0 1 2 2 2
  spline S118 degree 2 poles (52.5671, 28.9286) (52.5671, 28.6913) (52.8983, 28.4194) (53.3729, 28.3107) knots 0 0 0 1 2 2 2
  spline S119 degree 2 poles (53.3729, 28.3107) (53.6793, 28.2415) (54.2478, 28.108) (54.5741, 27.9943) knots 0 0 0 1 2 2 2
  spline S120 degree 2 poles (54.5741, 27.9943) (55.2068, 27.762) (55.8247, 26.9908) (55.8247, 26.3581) knots 0 0 0 1 2 2 2
  spline S121 degree 2 poles (55.8247, 26.3581) (55.8247, 25.4485) (54.3961, 24.3412) (53.1801, 24.3412) knots 0 0 0 1 2 2 2
  line L188 (39.8075, 5) -> (38.0814, 2.0867)
  line L189 (38.0814, 2.0867) -> (38.0814, 0)
  line L190 (38.0814, 0) -> (36.8254, 0)
  line L191 (36.8254, 0) -> (36.8254, 2.0259)
  line L192 (36.8254, 2.0259) -> (35.0709, 5)
  line L193 (35.0709, 5) -> (36.5012, 5)
  line L194 (36.5012, 5) -> (37.4777, 3.2172)
  line L195 (37.4777, 3.2172) -> (38.4218, 5)
  line L196 (38.4218, 5) -> (39.8075, 5)
  line L197 (58.6041, -7.5) -> (57.1536, -7.5)
  line L198 (57.1536, -7.5) -> (56.1892, -5.9076)
  line L199 (56.1892, -5.9076) -> (55.2046, -7.5)
  line L200 (55.2046, -7.5) -> (53.8148, -7.5)
  line L201 (53.8148, -7.5) -> (55.4396, -4.9838)
  line L202 (55.4396, -4.9838) -> (53.8797, -2.5)
  line L203 (53.8797, -2.5) -> (55.3302, -2.5)
  line L204 (55.3302, -2.5) -> (56.2338, -4.0113)
  line L205 (56.2338, -4.0113) -> (57.1617, -2.5)
  line L206 (57.1617, -2.5) -> (58.5515, -2.5)
  line L207 (58.5515, -2.5) -> (56.9834, -4.9311)
  line L208 (56.9834, -4.9311) -> (58.6041, -7.5)
  dimension "d18" = 10
  dimension "d19" = 50
  dimension "d20" = 10
  dimension "d21" = 10
  dimension "d22" = 50
  dimension "d23" = 10
  dimension "d24" = 7.5
  dimension "d25" = 7.5
  dimension "d26" = 7.5
  dimension "d27" = 7.5
  dimension "d28" = 7.5
  dimension "d29" = 7.5
  constraints: 44 end point, 16 coincident, 8 parallel, 7 midpoint, 4 horizontal, 4 perpendicular, 2 vertical, 1 point on line, 16 other
  measures "d18" distance of L36.start L36.end
  measures "d19" distance of L39.end L38.end
  measures "d20" distance of L38.end L37.end
  measures "d21" distance of L43.start L43.end
  measures "d22" distance of L46.end L45.end
  measures "d23" distance of L45.end L44.end
  measures "d24" distance of L68.end L66.start
  measures "d25" distance of L64.end L62.start
  measures "d26" distance of L60.end L58.start
  measures "d27" distance of L72.end L70.start
  measures "d28" distance of L76.end L74.start
  measures "d29" distance of L80.end L78.start
extrude "Extrusion3" cut sketch "Sketch2" against normal blind 1.25 contours L34 L191 L192 L193 L194 L195 L196 L188 L189 | L168 L169 L170 L43 | L43 L170 L171 L172 L165 L166 L167 L168 | S0 L82 L83 S1 S2 S3 S4 S5 S6 S7 S8 L84 L85 S9 S10 S11 S12 S13 S14 S15 | S16 L86 L87 S17 S18 S19 S20 S21 S22 S23 S24 L88 L89 S25 S26 S27 S28 S29 S30 S31 | L90 L91 L92 L93 L94 L95 L96 S32 S33 S34 L97 | S39 S40 S41 S42 | S51 S52 L101 L102 L103 S53 S54 | S59 L107 L108 S60 S61 S62 S63 S64 S65 S66 S67 L109 L110 S68 S69 S70 S71 S72 S73 S74 | L111 L112 L113 L114 L115 L116 L117 L118 L119 L120 | L121 L122 L123 L124 L125 L126 L127 L128 L129 | L130 L131 L132 L133 L134 L135 L136 L137 L138 L139 L140 L141 | L142 L143 L144 L145 L146 L147 L148 L149 L150 L151 | L152 L153 L154 L155 L156 L157 L158 L159 L160 L161 L162 L163 L164 | S75 S76 S77 S78 | S87 S88 S89 S90 | L173 L174 L175 L176 L177 L178 L179 S99 S100 S101 L180 | S106 L184 L185 S107 S108 S109 S110 S111 S112 S113 S114 L186 L187 S115 S116 S117 S118 S119 S120 S121 | L197 L198 L199 L200 L201 L202 L203 L204 L205 L206 L207 L208
fillet "Fillet1" radius 2.5 16 edges at (-75, 2.5, -37.5) (-75, 2.5, 37.5) (75, 2.5, 37.5) (75, 2.5, -37.5) (-53.75, 2.5, 12.5) (-35, 2.5, 15.5) (-16.25, 2.5, 18.5) (-58.75, 2.5, 12.5) (-40, 2.5, 15.5) (-21.25, 2.5, 18.5) (15, 2.5, 18.75) (33.75, 2.5, 20) (52.5, 2.5, 23.75) (22.5, 2.5, 18.75) (41.25, 2.5, 20) (60, 2.5, 23.75)
body "Solid1"
